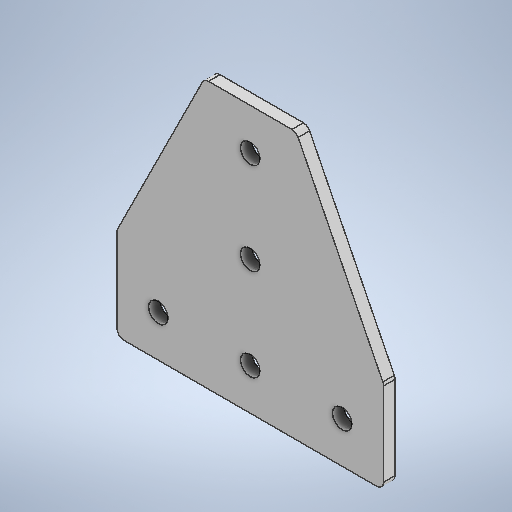
# Autodesk Inventor part: Connection_plate_T_120x120
Saved by Autodesk Inventor 2025.3 (Build 293356000, 356)
## iProperties
Created: 2026-05-31
Part Number: Connection_plate_T_120x120
Material: Generic
Document SubType Name: Modeling
Designer: louis
Density: 1 g/cm^3
Appearance: Default
Author: louis
Autodesk Inventor part; units mm, degrees
ref_plane "YZ Plane" through (0, 0, 0) normal (1, 0, 0) x (0, 1, 0)
ref_plane "XZ Plane" through (0, 0, 0) normal (0, 1, 0) x (-1, 0, 0)
ref_plane "XY Plane" through (0, 0, 0) normal (0, 0, 1) x (1, 0, 0)
sketch "Sketch1" plane through (0, 0, 0) normal (0, 0, 1) x (1, 0, 0)
  circle A0 centre (0, 0) radius 4.25
  circle A1 centre (-40, 0) radius 4.25
  circle A2 centre (40, 0) radius 4.25
  circle A3 centre (0, 80) radius 4.25
  circle A4 centre (0, 40) radius 4.25
  line L0 (0, 0) -> (0, 80) construction
  line L1 (-40, 0) -> (40, 0) construction
  line L2 (-58, 98) -> (58, 98)
  line L3 (58, 98) -> (58, -18)
  line L4 (58, -18) -> (-58, -18)
  line L5 (-58, -18) -> (-58, 98)
  line L6 (-58, 98) -> (58, -18) construction
  line L7 (58, 98) -> (-58, -18) construction
  line L8 (-58, 22) -> (-20, 98)
  line L9 (20, 98) -> (58, 22)
  dimension "d0" = 8.5
  dimension "d1" = 8.5
  dimension "d2" = 8.5
  dimension "d3" = 8.5
  dimension "d4" = 8.5
  dimension "d5" = 80
  dimension "d6" = 80
  dimension "d7" = 116
  dimension "d8" = 116
  dimension "d9" = 40
  dimension "d10" = 40
  dimension "d11" = 40
  constraints: 20 end point, 5 centre point, 4 midpoint, 4 point on line, 2 coincident, 2 horizontal, 2 parallel, 1 perpendicular, 1 symmetric about line, 1 vertical
  measures "d0" diameter of A0
  measures "d1" diameter of A4
  measures "d2" diameter of A3
  measures "d3" diameter of A2
  measures "d4" diameter of A1
  measures "d5" distance of L1.start L1.end
  measures "d6" distance of L0.start L0.end
  measures "d7" distance of L3.end L4.end
  measures "d8" distance of L2.end L3.end
  measures "d9" distance from line of L4 L8.start
  measures "d10" distance from line of L4 L9.end
  measures "d11" distance of L9.start L8.end
extrude "Extrusion1" add sketch "Sketch1" along normal mid plane 5 contours L2 L9 L3 L4 L5 L8
fillet "Fillet1" radius 3 6 edges at (-58, -18, 0) (-58, 22, 0) (20, 98, 0) (-20, 98, 0) (58, 22, 0) (58, -18, 0)
equation "\"d1\" = d0"
equation "\"d2\" = d0"
equation "\"d3\" = d0"
equation "\"d4\" = d0"
body "Solid1"
